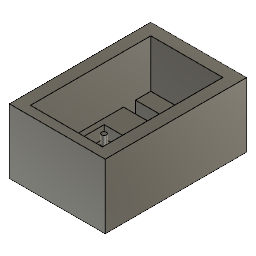
camera_flash mount v1 (Autodesk Fusion 360 design; units mm, degrees)
Autodesk Fusion 360 part; units mm, degrees
note: some values were not read from the file. Set by a fixed rule: which sketch regions a step uses.
sketch "Sketch1" plane through (0, 0, 0) normal (0, 0, 1) x (1, 0, 0)
  line L0 (0, 0) -> (0, 40)
  line L1 (0, 40) -> (40, 40)
  line L2 (40, 40) -> (40, 0)
  line L3 (40, 0) -> (0, 0)
  measures "d11" distance of L0.start
  measures "d14" distance of L0.start
  measures "d16" distance of L0.start
  measures "d27" distance of L0.start
  measures "d28" distance of L0.start
  measures "d33" distance of L0.start
  measures "d34" distance of L0.start
extrude "Extrude1" add sketch "Sketch1" along normal blind 7
sketch "Sketch2" plane through (0, 0, 7) normal (0, 0, 1) x (-1, 0, 0)
  line L0 (-40, 0) -> (-40, -40)
  line L1 (-40, -40) -> (0, -40)
  line L2 (0, -40) -> (0, 0)
  line L3 (0, 0) -> (-40, 0)
  line L4 (-32.8325, -7.75) -> (-7.3325, -7.75)
  line L5 (-7.3325, -7.75) -> (-7.3325, -32.25)
  line L6 (-7.3325, -32.25) -> (-32.8325, -32.25)
  line L7 (-32.8325, -32.25) -> (-32.8325, -7.75)
  line L8 (-32.8325, -7.75) -> (-7.3325, -32.25) construction
  line L9 (-7.3325, -7.75) -> (-32.8325, -32.25) construction
  dimension "d3" = 24.5
  dimension "d4" = 25.5
  measures "d4" distance of L2.end
extrude "Extrude2" cut sketch "Sketch2" against normal blind 5 contours L4 L5 L6 L7
sketch "Sketch3" plane through (0, 0, 7) normal (0, 0, 1) x (-1, 0, 0)
  line L0 (-7.3325, -7.75) -> (-7.3325, -32.25)
  line L1 (-7.3325, -32.25) -> (-32.8325, -32.25)
  line L2 (-32.8325, -32.25) -> (-32.8325, -7.75)
  line L3 (-32.8325, -7.75) -> (-7.3325, -7.75)
  line L4 (-40, 0) -> (-40, -40)
  line L5 (-40, -40) -> (0, -40)
  line L6 (0, -40) -> (0, 0)
  line L7 (0, 0) -> (-40, 0)
  line L8 (-7.3325, -7.75) -> (-7.3325, 0.0071)
  line L9 (-32.8325, -7.75) -> (-32.8325, 0.0018)
extrude "Extrude3" cut sketch "Sketch3" against normal blind 4 contours L3 L7 L8 L9
sketch "Sketch4" plane through (0, 0, 2) normal (0, 0, 1) x (-1, 0, 0)
  line L0 (-32.8325, -32.25) -> (-7.3325, -32.25)
  line L1 (-7.3325, -32.25) -> (-7.3325, -7.75)
  line L2 (-7.3325, -7.75) -> (-32.8325, -7.75)
  line L3 (-32.8325, -7.75) -> (-32.8325, -32.25)
  line L4 (-19.9972, -32) -> (-19.9972, -7.7499)
  line L5 (-7.3325, -20) -> (-32.8325, -20)
  line L6 (-23.9823, -7.75) -> (-23.9823, -14.25)
  line L7 (-23.9823, -14.25) -> (-7.3325, -14.25)
  line L8 (-23.9823, -14.25) -> (-32.8333, -14.25)
  line L9 (-19.9972, -14.25) -> (-19.9972, -18.25)
  line L10 (-23.9972, -14.25) -> (-15.9972, -14.25)
  line L11 (-15.9972, -14.25) -> (-15.9972, -22.25)
  line L12 (-15.9972, -22.25) -> (-23.9972, -22.25)
  line L13 (-23.9972, -22.25) -> (-23.9972, -14.25)
  line L14 (-23.9972, -14.25) -> (-15.9972, -22.25) construction
  line L15 (-15.9972, -14.25) -> (-23.9972, -22.25) construction
  dimension "d9" = 6.5
  dimension "d10" = 4
  dimension "d11" = 8
  measures "d11" distance of origin
extrude "Extrude4" cut sketch "Sketch4" against normal blind 5 contours L4 L5 L7 L8 L9 L10 L13 | L4 L5 L12 L13 | L4 L5 L11 L12 | L4 L5 L7 L9 L10 L11
sketch "Sketch5" plane through (0, 0, 2) normal (0, 0, 1) x (-1, 0, 0)
  line L0 (-15.9972, -14.25) -> (-15.9972, -22.25)
  line L1 (-15.9972, -22.25) -> (-23.9972, -22.25)
  line L2 (-23.9972, -22.25) -> (-23.9972, -14.25)
  line L3 (-23.9972, -14.25) -> (-15.9972, -14.25)
  line L4 (-32.8325, -32.25) -> (-7.3325, -32.25)
  line L5 (-7.3325, -32.25) -> (-7.3325, -7.75)
  line L6 (-7.3325, -7.75) -> (-32.8325, -7.75)
  line L7 (-32.8325, -7.75) -> (-32.8325, -32.25)
  line L8 (-20, -32) -> (-20.0825, -7.75)
  line L9 (-20, -32) -> (-20, -30)
  line L10 (-20, -30) -> (-30.4999, -30.0357)
  circle A0 centre (-30.4999, -30.0357) radius 1
  line L11 (-20, -30) -> (-9.5, -30)
  circle A1 centre (-9.5, -30) radius 1
  line L12 (-9.5, -30) -> (-9.5, -17.5)
  line L13 (-30.4999, -30.0357) -> (-30.5425, -17.5358)
  circle A2 centre (-9.5, -17.5) radius 1
  circle A3 centre (-30.5425, -17.5358) radius 1
  dimension "d14" = 10.5
  dimension "d15" = 2
  dimension "d16" = 10.5
  dimension "d17" = 2
  dimension "d18" = 12.5
  dimension "d19" = 12.5
  dimension "d20" = 2
  dimension "d21" = 2
  measures "d15" diameter of A0
  measures "d16" distance of origin
  measures "d17" diameter of A1
  measures "d19" distance of origin
  measures "d20" diameter of A2
  measures "d21" diameter of A3
extrude "Extrude5" add sketch "Sketch5" along normal blind 2 contours L10 A0 L13 | L10 A0 L13 | L11 A1 L12 | L11 A1 L12 | A2 | A3
sketch "Sketch6" plane through (0, 0, 7) normal (0, 0, 1) x (-1, 0, 0)
  line L0 (-32.8325, -32.25) -> (-32.8325, 0)
  line L1 (-32.8325, 0) -> (-40, 0)
  line L2 (-40, 0) -> (-40, -40)
  line L3 (-40, -40) -> (0, -40)
  line L4 (0, -40) -> (0, 0)
  line L5 (0, 0) -> (-7.3325, 0)
  line L6 (-7.3325, 0) -> (-7.3325, -32.25)
  line L7 (-7.3325, -32.25) -> (-32.8325, -32.25)
  line L8 (-40, 0) -> (0, 0)
  line L9 (-20, -40) -> (-20, 0)
  line L10 (-20, -40) -> (-20, -36.5)
  line L11 (-20, -36.5) -> (-36, -36.5)
  line L12 (-20, -36.5) -> (-4, -36.5)
  circle A0 centre (-36, -36.5) radius 2.5
  circle A1 centre (-4, -36.5) radius 2.5
  line L13 (-36, -36.5) -> (-36, -6.5)
  line L14 (-4, -36.5) -> (-4, -6.5)
  circle A2 centre (-36, -6.5) radius 2.5
  circle A3 centre (-4, -6.5) radius 2.5
  dimension "d24" = 3.5
  dimension "d25" = 5
  dimension "d26" = 5
  dimension "d27" = 30
  dimension "d28" = 30
  dimension "d29" = 5
  dimension "d30" = 5
  measures "d25" diameter of A0
  measures "d26" diameter of A1
  measures "d27" distance of L4.end
  measures "d29" diameter of A2
  measures "d30" diameter of A3
extrude "Extrude6" cut sketch "Sketch6" against normal blind 7 contours L11 A0 L13 | L11 A0 L13 | L12 A1 L14 | L12 A1 L14 | A2 | A3
sketch "Sketch7" plane through (0, 0, 7) normal (0, 0, 1) x (-1, 0, 0)
  circle A0 centre (-4, -36.5) radius 2.5
  circle A1 centre (-36, -36.5) radius 2.5
  circle A2 centre (-4, -6.5) radius 2.5
  circle A3 centre (-36, -6.5) radius 2.5
  line L0 (-32.8325, -32.25) -> (-32.8325, 0)
  line L1 (-32.8325, 0) -> (-40, 0)
  line L2 (-40, 0) -> (-40, -40)
  line L3 (-40, -40) -> (0, -40)
  line L4 (0, -40) -> (0, 0)
  line L5 (0, 0) -> (-7.3325, 0)
  line L6 (-7.3325, 0) -> (-7.3325, -32.25)
  line L7 (-7.3325, -32.25) -> (-32.8325, -32.25)
  line L8 (-15.9972, -22.25) -> (-23.9972, -14.25)
  line L9 (-23.9972, -14.25) -> (-23.9972, -22.25)
  line L10 (-23.9972, -22.25) -> (-15.9972, -14.25)
  line L11 (-24.2472, -14) -> (-15.7472, -14)
  line L12 (-15.7472, -14) -> (-15.7472, -22.5)
  line L13 (-15.7472, -22.5) -> (-24.2472, -22.5)
  line L14 (-24.2472, -22.5) -> (-24.2472, -14)
  line L15 (-24.2472, -14) -> (-15.7472, -22.5) construction
  line L16 (-15.7472, -14) -> (-24.2472, -22.5) construction
  dimension "d33" = 8.5
  dimension "d34" = 8.5
  measures "d33" distance of L4.end
extrude "Extrude7" cut sketch "Sketch7" against normal blind 20 contours L8 L9 L10 | L11 L12 L13 L14
sketch "Sketch8" plane through (0, 0, 2) normal (0, 0, 1) x (-1, 0, 0)
  line L0 (-15.7472, -14) -> (-15.7472, -22.5)
  line L1 (-15.7472, -22.5) -> (-24.2472, -22.5)
  line L2 (-24.2472, -22.5) -> (-24.2472, -14)
  line L3 (-24.2472, -14) -> (-15.7472, -14)
  circle A0 centre (-9.5, -17.5) radius 1
  circle A1 centre (-30.4999, -30.0357) radius 1
  circle A2 centre (-30.5425, -17.5358) radius 1
  circle A3 centre (-9.5, -30) radius 1
  line L4 (-32.8325, -32.25) -> (-7.3325, -32.25)
  line L5 (-7.3325, -32.25) -> (-7.3325, -7.75)
  line L6 (-7.3325, -7.75) -> (-32.8325, -7.75)
  line L7 (-32.8325, -7.75) -> (-32.8325, -32.25)
  line L8 (-15.7472, -27.8448) -> (-24.2472, -27.8448)
  line L9 (-24.2472, -27.8448) -> (-24.2472, -17.1552)
  line L10 (-24.2472, -17.1552) -> (-15.7472, -17.1552)
  line L11 (-15.7472, -17.1552) -> (-15.7472, -27.8448)
  line L12 (-15.7472, -27.8448) -> (-24.2472, -17.1552) construction
  line L13 (-24.2472, -27.8448) -> (-15.7472, -17.1552) construction
extrude "Extrude8" cut sketch "Sketch8" against normal blind 20 contours L1 L8 L9 L11
sketch "Sketch9" plane through (0, 0, 2) normal (0, 0, 1) x (-1, 0, 0)
  line L0 (-24.2472, -27.8448) -> (-24.2472, -14)
  line L1 (-24.2472, -14) -> (-15.7472, -14)
  line L2 (-15.7472, -14) -> (-15.7472, -27.8448)
  line L3 (-15.7472, -27.8448) -> (-24.2472, -27.8448)
  circle A0 centre (-9.5, -17.5) radius 1
  circle A1 centre (-30.4999, -30.0357) radius 1
  circle A2 centre (-30.5425, -17.5358) radius 1
  circle A3 centre (-9.5, -30) radius 1
  line L4 (-32.8325, -32.25) -> (-7.3325, -32.25)
  line L5 (-7.3325, -32.25) -> (-7.3325, -7.75)
  line L6 (-7.3325, -7.75) -> (-32.8325, -7.75)
  line L7 (-32.8325, -7.75) -> (-32.8325, -32.25)
  line L8 (-15.7472, -30.1146) -> (-24.2472, -30.1146)
  line L9 (-24.2472, -30.1146) -> (-24.2472, -25.575)
  line L10 (-24.2472, -25.575) -> (-15.7472, -25.575)
  line L11 (-15.7472, -25.575) -> (-15.7472, -30.1146)
  line L12 (-15.7472, -30.1146) -> (-24.2472, -25.575) construction
  line L13 (-24.2472, -30.1146) -> (-15.7472, -25.575) construction
extrude "Extrude9" cut sketch "Sketch9" against normal blind 20 contours L3 L8 L9 L11
sketch "Sketch10" plane through (0, 0, 2) normal (0, 0, 1) x (-1, 0, 0)
  line L0 (-32.8325, -32.25) -> (-7.3325, -32.25)
  line L1 (-7.3325, -32.25) -> (-7.3325, -7.75)
  line L2 (-7.3325, -7.75) -> (-32.8325, -7.75)
  line L3 (-32.8325, -7.75) -> (-32.8325, -32.25)
  circle A0 centre (-9.5, -30) radius 1
  circle A1 centre (-30.5425, -17.5358) radius 1
  circle A2 centre (-30.4999, -30.0357) radius 1
  circle A3 centre (-9.5, -17.5) radius 1
  line L4 (-15.7472, -14) -> (-15.7472, -30.1146)
  line L5 (-15.7472, -30.1146) -> (-24.2472, -30.1146)
  line L6 (-24.2472, -30.1146) -> (-24.2472, -14)
  line L7 (-24.2472, -14) -> (-15.7472, -14)
  line L8 (-24.2472, -30.1146) -> (-28, -30.1146)
  line L9 (-28, -30.1146) -> (-28, -26)
  line L10 (-28, -26) -> (-24.2472, -26.029)
extrude "Extrude10" cut sketch "Sketch10" against normal blind 20 contours L6 L8 L9 L10
sketch "Sketch11" plane through (0, 0, 4) normal (0, 0, 1) x (-1, 0, 0)
  circle A0 centre (-9.5, -30) radius 1
  circle A1 centre (-9.5, -30) radius 1
extrude "Extrude11" add sketch "Sketch11" along normal blind 2
sketch "Sketch12" plane through (0, 0, 4) normal (0, 0, 1) x (-1, 0, 0)
  circle A0 centre (-9.5, -17.5) radius 1
  circle A1 centre (-9.5, -17.5) radius 1
extrude "Extrude12" add sketch "Sketch12" along normal blind 2
sketch "Sketch13" plane through (0, 0, 4) normal (0, 0, 1) x (-1, 0, 0)
  circle A0 centre (-30.4999, -30.0357) radius 1
  circle A1 centre (-30.4999, -30.0357) radius 1
extrude "Extrude13" add sketch "Sketch13" along normal blind 2
sketch "Sketch14" plane through (0, 0, 4) normal (0, 0, 1) x (-1, 0, 0)
  circle A0 centre (-30.5425, -17.5358) radius 1
  circle A1 centre (-30.5425, -17.5358) radius 1
extrude "Extrude14" add sketch "Sketch14" along normal blind 2
sketch "Sketch15" plane through (0, 0, 7) normal (0, 0, 1) x (-1, 0, 0)
  circle A0 centre (-4, -36.5) radius 2.5
  circle A1 centre (-36, -36.5) radius 2.5
  circle A2 centre (-4, -6.5) radius 2.5
  circle A3 centre (-36, -6.5) radius 2.5
  line L0 (-32.8325, -32.25) -> (-32.8325, 0)
  line L1 (-32.8325, 0) -> (-40, 0)
  line L2 (-40, 0) -> (-40, -40)
  line L3 (-40, -40) -> (0, -40)
  line L4 (0, -40) -> (0, 0)
  line L5 (0, 0) -> (-7.3325, 0)
  line L6 (-7.3325, 0) -> (-7.3325, -32.25)
  line L7 (-7.3325, -32.25) -> (-32.8325, -32.25)
  circle A4 centre (-4, -36.5) radius 2.5
extrude "Extrude15" add sketch "Sketch15" against normal blind 5 contours A0 A4
sketch "Sketch16" plane through (0, 0, 2) normal (0, 0, -1) x (1, 0, 0)
  circle A0 centre (4, -36.5) radius 2.5
  circle A1 centre (4, -36.5) radius 2.5
extrude "Extrude16" add sketch "Sketch16" along normal blind 2
sketch "Sketch17" plane through (0, 0, 0) normal (0, 0, 1) x (1, 0, 0)
  circle A0 centre (4, 6.5) radius 2.5
  circle A1 centre (4, 6.5) radius 2.5
  circle A2 centre (4, 6.5) radius 2.5
extrude "Extrude17" add sketch "Sketch17" along normal blind 7
sketch "Sketch18" plane through (0, 0, 7) normal (0, 0, 1) x (-1, 0, 0)
  circle A0 centre (-36, -36.5) radius 2.5
  circle A1 centre (-36, -6.5) radius 2.5
  line L0 (-32.8325, -32.25) -> (-32.8325, 0)
  line L1 (-32.8325, 0) -> (-40, 0)
  line L2 (-40, 0) -> (-40, -40)
  line L3 (-40, -40) -> (0, -40)
  line L4 (0, -40) -> (0, 0)
  line L5 (0, 0) -> (-7.3325, 0)
  line L6 (-7.3325, 0) -> (-7.3325, -32.25)
  line L7 (-7.3325, -32.25) -> (-32.8325, -32.25)
  circle A2 centre (-36, -36.5) radius 2.5
extrude "Extrude18" add sketch "Sketch18" against normal blind 7 contours A0 A2
sketch "Sketch19" plane through (0, 0, 7) normal (0, 0, 1) x (-1, 0, 0)
  circle A0 centre (-36, -6.5) radius 2.5
  line L0 (-32.8325, -32.25) -> (-32.8325, 0)
  line L1 (-32.8325, 0) -> (-40, 0)
  line L2 (-40, 0) -> (-40, -40)
  line L3 (-40, -40) -> (0, -40)
  line L4 (0, -40) -> (0, 0)
  line L5 (0, 0) -> (-7.3325, 0)
  line L6 (-7.3325, 0) -> (-7.3325, -32.25)
  line L7 (-7.3325, -32.25) -> (-32.8325, -32.25)
  circle A1 centre (-36, -6.5) radius 2.5
extrude "Extrude19" add sketch "Sketch19" against normal blind 7 contours A0 A1
sketch "Sketch20" plane through (0, 0, 0) normal (0, 0, 1) x (1, 0, 0)
  line L0 (40, 40) -> (0, 40)
  line L1 (0, 40) -> (0, 61.8124)
  line L2 (0, 61.8124) -> (40, 61.8124)
  line L3 (40, 61.8124) -> (40, 40)
  line L4 (40, 40) -> (0, 61.8124) construction
  line L5 (0, 40) -> (40, 61.8124) construction
extrude "Extrude20" add sketch "Sketch20" along normal blind 7
sketch "Sketch21" plane through (0, 0, 7) normal (0, 0, 1) x (-1, 0, 0)
  line L0 (-32.8325, -32.25) -> (-32.8325, 0)
  line L1 (-32.8325, 0) -> (-40, 0)
  line L2 (-40, 0) -> (-40, -61.8124)
  line L3 (-40, -61.8124) -> (0, -61.8124)
  line L4 (0, -61.8124) -> (0, 0)
  line L5 (0, 0) -> (-7.3325, 0)
  line L6 (-7.3325, 0) -> (-7.3325, -32.25)
  line L7 (-7.3325, -32.25) -> (-32.8325, -32.25)
  line L8 (-35, -42.6061) -> (-5, -42.6061)
  line L9 (-5, -42.6061) -> (-5, -47.6061)
  line L10 (-5, -47.6061) -> (-35, -47.6061)
  line L11 (-35, -47.6061) -> (-35, -42.6061)
  line L12 (-35, -42.6061) -> (-5, -47.6061) construction
  line L13 (-5, -42.6061) -> (-35, -47.6061) construction
  dimension "d63" = 5
  dimension "d64" = 30
  measures "d64" distance of L4.end
extrude "Extrude21" cut sketch "Sketch21" against normal blind 7 contours L8 L9 L10 L11
sketch "Sketch22" plane through (0, 0, 7) normal (0, 0, 1) x (-1, 0, 0)
  line L0 (-5, -42.6061) -> (-5, -47.6061)
  line L1 (-5, -47.6061) -> (-35, -47.6061)
  line L2 (-35, -47.6061) -> (-35, -42.6061)
  line L3 (-35, -42.6061) -> (-5, -42.6061)
  line L4 (-32.8325, -32.25) -> (-32.8325, 0)
  line L5 (-32.8325, 0) -> (-40, 0)
  line L6 (-40, 0) -> (-40, -61.8124)
  line L7 (-40, -61.8124) -> (0, -61.8124)
  line L8 (0, -61.8124) -> (0, 0)
  line L9 (0, 0) -> (-7.3325, 0)
  line L10 (-7.3325, 0) -> (-7.3325, -32.25)
  line L11 (-7.3325, -32.25) -> (-32.8325, -32.25)
  line L12 (-20, -45) -> (-20, -56)
  line L13 (-20, -56) -> (-20, -61.8124)
  line L14 (-40, -59) -> (0, -59)
  line L15 (0, -59) -> (0, -64.6248)
  line L16 (0, -64.6248) -> (-40, -64.6248)
  line L17 (-40, -64.6248) -> (-40, -59)
  line L18 (-40, -59) -> (0, -64.6248) construction
  line L19 (0, -59) -> (-40, -64.6248) construction
  dimension "d67" = 5.6248
extrude "Extrude22" cut sketch "Sketch22" against normal blind 7 contours L6 L7 L13 L14 L17 | L7 L8 L13 L14 L15
sketch "Sketch23" plane through (0, 0, 7) normal (0, 0, 1) x (-1, 0, 0)
  line L0 (-40, -59) -> (0, -59)
  line L1 (0, -59) -> (0, 0)
  line L2 (0, 0) -> (-7.3325, 0)
  line L3 (-7.3325, 0) -> (-7.3325, -32.25)
  line L4 (-7.3325, -32.25) -> (-32.8325, -32.25)
  line L5 (-32.8325, -32.25) -> (-32.8325, 0)
  line L6 (-32.8325, 0) -> (-40, 0)
  line L7 (-40, 0) -> (-40, -59)
  line L8 (-5, -42.6061) -> (-5, -47.6061)
  line L9 (-5, -47.6061) -> (-35, -47.6061)
  line L10 (-35, -47.6061) -> (-35, -42.6061)
  line L11 (-35, -42.6061) -> (-5, -42.6061)
  circle A0 centre (-4, -55) radius 2.5
  circle A1 centre (-37, -55) radius 2.5
  circle A2 centre (-37, -4) radius 2.5
  circle A3 centre (-3.5618, -3.875) radius 2.5
  dimension "d70" = 5
  dimension "d71" = 5
  dimension "d72" = 5
  dimension "d73" = 5
  measures "d70" diameter of A0
  measures "d71" diameter of A1
  measures "d72" diameter of A2
  measures "d73" diameter of A3
extrude "Extrude23" add sketch "Sketch23" along normal blind 5 contours A0 | A1 | A2 | A3
sketch "Sketch24" plane through (0, 0, 12) normal (0, 0, 1) x (-1, 0, 0)
  circle A0 centre (-4, -55) radius 2.5
  circle A1 centre (-4, -55) radius 1
  circle A2 centre (-37, -55) radius 1
extrude "Extrude24" cut sketch "Sketch24" against normal blind 3 contours A1 | A2
sketch "Sketch25" plane through (0, 0, 12) normal (0, 0, 1) x (-1, 0, 0)
  circle A0 centre (-3.5618, -3.875) radius 2.5
  circle A1 centre (-3.5618, -3.875) radius 1
  circle A2 centre (-37, -4) radius 1
  dimension "d78" = 2
  measures "d78" diameter of A1
extrude "Extrude25" cut sketch "Sketch25" against normal blind 3 contours A1 | A2
sketch "Sketch26" plane through (0, 0, 0) normal (0, 0, -1) x (1, 0, 0)
  line L0 (0, -59) -> (40, -59)
  line L1 (40, -59) -> (40, 0)
  line L2 (40, 0) -> (0, 0)
  line L3 (0, 0) -> (0, -59)
  line L4 (5, -47.6061) -> (5, -42.6061)
  line L5 (5, -42.6061) -> (35, -42.6061)
  line L6 (35, -42.6061) -> (35, -47.6061)
  line L7 (35, -47.6061) -> (5, -47.6061)
  line L8 (28, -30.1146) -> (15.7472, -30.1146)
  line L9 (15.7472, -30.1146) -> (15.7472, -14)
  line L10 (15.7472, -14) -> (24.2472, -14)
  line L11 (24.2472, -14) -> (24.2472, -26.029)
  line L12 (24.2472, -26.029) -> (28, -26)
  line L13 (28, -26) -> (28, -30.1146)
  line L14 (30.5, -55.6314) -> (9.5, -55.6314)
  line L15 (9.5, -55.6314) -> (9.5, -34.6314)
  line L16 (9.5, -34.6314) -> (30.5, -34.6314)
  line L17 (30.5, -34.6314) -> (30.5, -55.6314)
  line L18 (30.5, -55.6314) -> (9.5, -34.6314) construction
  line L19 (9.5, -55.6314) -> (30.5, -34.6314) construction
  dimension "d81" = 21
  dimension "d82" = 21
  measures "d81" distance of L2.end
extrude "Extrude26" cut sketch "Sketch26" against normal blind 2 contours L7 L14 L15 L17 | L5 L15 L16 L17
extrude "Extrude27" cut 1 faces at (35.013, 4.1739, 12) along direction (0, 0, -1) blind 5
extrude "Extrude28" cut 1 faces at (36.9751, 4.3324, 9) along direction (0, 0, -1) blind 2
extrude "Extrude29" cut 1 faces at (1.5748, 4.0489, 12) along direction (0, 0, -1) blind 5
extrude "Extrude30" cut 1 faces at (3.9958, 3.666, 9) along direction (0, 0, -1) blind 2
extrude "Extrude31" cut 1 faces at (2.013, 55.1739, 12) along direction (0, 0, -1) blind 5
extrude "Extrude32" cut 1 faces at (4.6415, 54.7287, 9) along direction (0, 0, -1) blind 2
extrude "Extrude33" cut 1 faces at (35.013, 55.1739, 12) along direction (0, 0, -1) blind 5
extrude "Extrude34" cut 1 faces at (37.4221, 54.7901, 9) along direction (0, 0, -1) blind 2
sketch "Sketch27" plane through (0, 0, 3) normal (0, 0, 1) x (-1, 0, 0)
  line L0 (-7.3325, -7.75) -> (-7.3325, 0)
  line L1 (-7.3325, 0) -> (-32.8325, 0)
  line L2 (-32.8325, 0) -> (-32.8325, -7.75)
  line L3 (-32.8325, -7.75) -> (-7.3325, -7.75)
  line L4 (-7.3325, -3.875) -> (-32.8325, -3.875)
  line L5 (-7.3325, -3.875) -> (-7.3325, 0)
  line L6 (-7.3325, 0) -> (-32.8325, 0)
  line L7 (-32.8325, 0) -> (-32.8325, -3.875)
extrude "Extrude35" add sketch "Sketch27" along normal blind 4 contours L0 L1 L2 L4 L5 L6 L7
sketch "Sketch28" plane through (0, 0, 7) normal (0, 0, 1) x (-1, 0, 0)
  line L0 (0, 0) -> (-40, 0)
  line L1 (-40, 0) -> (-40, -59)
  line L2 (-40, -59) -> (0, -59)
  line L3 (0, -59) -> (0, 0)
  line L4 (-32.8325, -3.875) -> (-7.3325, -3.875)
  line L5 (-7.3325, -3.875) -> (-7.3325, -32.25)
  line L6 (-7.3325, -32.25) -> (-32.8325, -32.25)
  line L7 (-32.8325, -32.25) -> (-32.8325, -3.875)
  line L8 (-5, -42.6061) -> (-5, -47.6061)
  line L9 (-5, -47.6061) -> (-35, -47.6061)
  line L10 (-35, -47.6061) -> (-35, -42.6061)
  line L11 (-35, -42.6061) -> (-5, -42.6061)
  line L12 (0, -59) -> (-40, -59)
  line L13 (-40, -59) -> (-40, -54)
  line L14 (-40, -54) -> (0, -54)
  line L15 (0, -54) -> (0, -59)
  dimension "d103" = 5
extrude "Extrude36" add sketch "Sketch28" along normal blind 20 contours L1 L2 L3 L12 L13 L14 L15
sketch "Sketch29" plane through (0, 0, 7) normal (0, 0, 1) x (-1, 0, 0)
  line L0 (-5, -42.6061) -> (-5, -47.6061)
  line L1 (-5, -47.6061) -> (-35, -47.6061)
  line L2 (-35, -47.6061) -> (-35, -42.6061)
  line L3 (-35, -42.6061) -> (-5, -42.6061)
  line L4 (-32.8325, -3.875) -> (-7.3325, -3.875)
  line L5 (-7.3325, -3.875) -> (-7.3325, -32.25)
  line L6 (-7.3325, -32.25) -> (-32.8325, -32.25)
  line L7 (-32.8325, -32.25) -> (-32.8325, -3.875)
  line L8 (-40, -54) -> (0, -54)
  line L9 (0, -54) -> (0, 0)
  line L10 (0, 0) -> (-40, 0)
  line L11 (-40, 0) -> (-40, -54)
  line L12 (-40, -54) -> (-35, -54)
  line L13 (-35, -54) -> (-35, 0)
  line L14 (-35, 0) -> (-40, 0)
  line L15 (-40, 0) -> (-40, -54)
extrude "Extrude37" add sketch "Sketch29" along normal blind 20 contours L2 L8 L10 L11 L12 L13 L14 L15
sketch "Sketch30" plane through (0, 0, 7) normal (0, 0, 1) x (-1, 0, 0)
  line L0 (-35, 0) -> (-35, -42.6061)
  line L1 (-35, -42.6061) -> (-5, -42.6061)
  line L2 (-5, -42.6061) -> (-5, -47.6061)
  line L3 (-5, -47.6061) -> (-35, -47.6061)
  line L4 (-35, -47.6061) -> (-35, -54)
  line L5 (-35, -54) -> (0, -54)
  line L6 (0, -54) -> (0, 0)
  line L7 (0, 0) -> (-35, 0)
  line L8 (-32.8325, -3.875) -> (-7.3325, -3.875)
  line L9 (-7.3325, -3.875) -> (-7.3325, -32.25)
  line L10 (-7.3325, -32.25) -> (-32.8325, -32.25)
  line L11 (-32.8325, -32.25) -> (-32.8325, -3.875)
  line L12 (0, -54) -> (-5, -54)
  line L13 (-5, -54) -> (-5, 0)
  line L14 (-5, 0) -> (0, 0)
  line L15 (0, 0) -> (0, -54)
extrude "Extrude38" add sketch "Sketch30" along normal blind 20 contours L2 L5 L6 L7 L12 L13 L14 L15
sketch "Sketch31" plane through (0, 0, 7) normal (0, 0, 1) x (-1, 0, 0)
  line L0 (-5, -42.6061) -> (-5, 0)
  line L1 (-5, 0) -> (-35, 0)
  line L2 (-35, 0) -> (-35, -42.6061)
  line L3 (-35, -42.6061) -> (-5, -42.6061)
  line L4 (-32.8325, -3.875) -> (-7.3325, -3.875)
  line L5 (-7.3325, -3.875) -> (-7.3325, -32.25)
  line L6 (-7.3325, -32.25) -> (-32.8325, -32.25)
  line L7 (-32.8325, -32.25) -> (-32.8325, -3.875)
  line L8 (-5, 0) -> (-35, 0)
  line L9 (-35, 0) -> (-35, -3.8534)
  line L10 (-35, -3.8534) -> (-5, -3.8534)
  line L11 (-5, -3.8534) -> (-5, 0)
extrude "Extrude39" add sketch "Sketch31" along normal blind 20 contours L0 L1 L2 L8 L9 L10 L11
